Autodesk Fusion 360 part; units mm, degrees
(part 5 of 11)
  line L412 (61.967, 22.9336) -> (61.967, 23.934)
  line L413 (47.167, 19.8345) -> (47.167, 22.9336)
  line L414 (61.967, 19.8345) -> (62.768, 19.8345)
  line L415 (47.967, 23.934) -> (61.967, 23.934)
  line L416 (47.967, 22.9336) -> (47.967, 23.934)
  line L417 (47.967, 22.9336) -> (47.167, 22.9336)
  line L418 (47.167, 19.8345) -> (47.967, 19.8345)
  line L419 (62.768, 22.9336) -> (61.967, 22.9336)
  line L420 (88.162, 4.8841) -> (88.162, 3.8837)
  line L421 (83.685, 14.6338) -> (83.685, 14.0343)
  line L422 (88.961, 3.8837) -> (88.961, 0.7845)
  line L423 (88.162, 3.8837) -> (88.961, 3.8837)
  line L424 (88.162, 0.7845) -> (88.961, 0.7845)
  line L425 (88.162, 3.8837) -> (88.162, 4.8841)
  line L426 (88.961, 0.7845) -> (88.162, 0.7845)
  line L427 (83.685, 14.0343) -> (83.685, 14.6338)
  line L428 (88.961, 3.8837) -> (88.162, 3.8837)
  line L429 (88.961, 0.7845) -> (88.961, 3.8837)
  line L430 (43.205, 95.6582) -> (57.206, 95.6582)
  line L431 (82.162, 10.1634) -> (82.162, 14.6338)
  line L432 (77.137, 9.1836) -> (80.435, 9.1836)
  line L433 (80.435, 10.1634) -> (82.162, 10.1634)
  line L434 (74.161, 3.8837) -> (73.362, 3.8837)
  line L435 (80.435, 9.1836) -> (77.137, 9.1836)
  line L436 (47.681, 62.034) -> (33.68, 62.034)
  line L437 (82.887, 10.9337) -> (82.887, 14.0343)
  line L438 (83.685, 14.6338) -> (82.162, 14.6338)
  line L439 (75.411, 16.4335) -> (75.411, 10.1634)
  line L440 (83.685, 10.9337) -> (83.685, 9.9333)
  line L441 (77.137, 9.1836) -> (77.137, 10.1634)
  line L442 (74.161, 4.8841) -> (74.161, 3.8837)
  line L443 (73.362, 3.8837) -> (74.161, 3.8837)
  line L444 (75.411, 10.1634) -> (75.411, 16.4335)
  line L445 (74.161, 3.8837) -> (74.161, 4.8841)
  line L446 (82.162, 14.6338) -> (82.162, 10.1634)
  line L447 (73.362, 3.8837) -> (73.362, 0.7845)
  line L448 (73.362, 0.7845) -> (74.161, 0.7845)
  line L449 (77.137, 10.1634) -> (77.137, 9.1836)
  line L450 (77.137, 10.1634) -> (75.411, 10.1634)
  line L451 (162.267, 71.1844) -> (162.267, 76.9844)
  line L452 (23.867, 14.0343) -> (24.668, 14.0343)
  line L453 (-118.7201, 61.0336) -> (-118.7201, 62.034)
  line L454 (243.23, 81.084) -> (243.23, 80.0836)
  line L455 (238.979, 80.0836) -> (238.182, 80.0836)
  line L456 (162.267, 99.7592) -> (162.267, 105.5592)
  line L457 (161.467, 96.6592) -> (161.467, 99.7592)
  line L458 (28.117, 10.9337) -> (28.117, 14.0343)
  line L459 (177.068, 68.0838) -> (177.068, 71.1844)
  line L460 (243.23, 76.9844) -> (242.429, 76.9844)
  line L461 (177.068, 71.1844) -> (176.267, 71.1844)
  line L462 (-123.769, 62.034) -> (-123.769, 61.0336)
  line L463 (26.536, 4.8841) -> (26.536, 3.8837)
  line L464 (-123.769, 57.9344) -> (-123.769, 52.1344)
  line L465 (212.856, -9.8664) -> (212.856, -8.8866)
  line L466 (258.029, 76.9844) -> (257.232, 76.9844)
  line L467 (-118.7201, 57.9344) -> (-119.5191, 57.9344)
  line L468 (161.467, 96.6592) -> (162.267, 96.6592)
  line L469 (177.068, 76.9844) -> (177.068, 80.0836)
  line L470 (209.607, -8.1163) -> (209.607, -9.1167)
  line L471 (23.867, 9.9333) -> (23.867, 10.9337)
  line L472 (224.18, 81.084) -> (238.182, 81.084)
  line L473 (-118.7201, 52.1344) -> (-118.7201, 57.9344)
  line L474 (209.607, -4.4162) -> (209.607, -5.0157)
  line L475 (158.018, 99.7592) -> (158.018, 96.6592)
  line L476 (161.467, 108.6602) -> (162.267, 108.6602)
  line L477 (26.536, 3.8837) -> (25.737, 3.8837)
  line L478 (257.232, 81.084) -> (243.23, 81.084)
  line L479 (224.18, 42.984) -> (238.182, 42.984)
  line L480 (210.404, -8.1163) -> (209.607, -8.1163)
  line L481 (-118.7201, 52.1344) -> (-119.5191, 52.1344)
  line L482 (157.217, 105.5592) -> (158.018, 105.5592)
  line L483 (24.668, 14.0343) -> (23.867, 14.0343)
  line L484 (-28.233, 23.934) -> (-14.233, 23.934)
  line L485 (238.979, 80.0836) -> (238.979, 76.9844)
  line L486 (23.867, 10.9337) -> (24.668, 10.9337)
  line L487 (158.018, 105.5592) -> (157.217, 105.5592)
  line L488 (216.154, -9.8664) -> (212.856, -9.8664)
  line L489 (243.23, 80.0836) -> (242.429, 80.0836)
  line L490 (257.232, 71.1844) -> (257.232, 76.9844)
  line L491 (25.737, 0.7845) -> (26.536, 0.7845)
  line L492 (-123.769, 61.0336) -> (-122.97, 61.0336)
  line L493 (-118.7201, 49.0338) -> (-118.7201, 48.0333)
  line L494 (211.131, -4.4162) -> (209.607, -4.4162)
  line L495 (238.182, 76.9844) -> (238.979, 76.9844)
  line L496 (243.23, 76.9844) -> (243.23, 71.1844)
  line L497 (157.217, 96.6592) -> (158.018, 96.6592)
  line L498 (177.068, 80.0836) -> (176.267, 80.0836)
  line L499 (209.607, -8.1163) -> (210.404, -8.1163)
  line L500 (-118.7201, 57.9344) -> (-118.7201, 52.1344)
  line L501 (210.404, -5.0157) -> (209.607, -5.0157)
  line L502 (177.068, 76.9844) -> (176.267, 76.9844)
  line L503 (162.267, 68.0838) -> (162.267, 67.0833)
  line L504 (176.267, 67.0833) -> (176.267, 68.0838)
  line L505 (242.429, 80.0836) -> (242.429, 76.9844)
  line L506 (23.356, 71.1844) -> (23.356, 68.0838)
  line L507 (177.068, 80.0836) -> (177.068, 76.9844)
  line L508 (-122.97, 49.0338) -> (-123.769, 49.0338)
  line L509 (161.467, 105.5592) -> (162.267, 105.5592)
  line L510 (210.404, -8.1163) -> (210.404, -5.0157)
  line L511 (158.018, 105.5592) -> (158.018, 108.6602)
  line L512 (209.607, -9.1167) -> (209.607, -8.1163)
  line L513 (-123.769, 48.0333) -> (-123.769, 49.0338)
  line L514 (258.029, 76.9844) -> (258.029, 80.0836)
  line L515 (158.018, 108.6602) -> (157.217, 108.6602)
  line L516 (238.182, 80.0836) -> (238.979, 80.0836)
  line L517 (24.155, 68.0838) -> (24.155, 67.0833)
  line L518 (-119.5191, 52.1344) -> (-118.7201, 52.1344)
  line L519 (176.267, 76.9844) -> (177.068, 76.9844)
  line L520 (238.979, 76.9844) -> (238.182, 76.9844)
  line L521 (-122.97, 52.1344) -> (-122.97, 49.0338)
  line L522 (176.267, 80.0836) -> (177.068, 80.0836)
  line L523 (210.404, -5.0157) -> (210.404, -8.1163)
  line L524 (24.668, 14.0343) -> (24.668, 10.9337)
  line L525 (177.068, 71.1844) -> (177.068, 68.0838)
  line L526 (242.429, 76.9844) -> (242.429, 80.0836)
  line L527 (162.267, 96.6592) -> (162.267, 95.6582)
  line L528 (211.131, -8.8866) -> (212.856, -8.8866)
  line L529 (24.155, 67.0833) -> (24.155, 68.0838)
  line L530 (212.856, -8.8866) -> (212.856, -9.8664)
  line L531 (-119.5191, 61.0336) -> (-118.7201, 61.0336)
  line L532 (-30.902, 0.1836) -> (8.724, 0.1836)
  line L533 (25.737, 0.7845) -> (25.737, 3.8837)
  line L534 (176.267, 68.0838) -> (176.267, 67.0833)
  line L535 (243.23, 80.0836) -> (243.23, 81.084)
  line L536 (24.155, 71.1844) -> (24.155, 76.9844)
  line L537 (-123.769, 49.0338) -> (-123.769, 48.0333)
  line L538 (23.356, 76.9844) -> (23.356, 80.0836)
  line L539 (258.029, 80.0836) -> (258.029, 76.9844)
  line L540 (-122.97, 52.1344) -> (-123.769, 52.1344)
  line L541 (26.536, 0.7845) -> (25.737, 0.7845)
  line L542 (25.737, 3.8837) -> (26.536, 3.8837)
  line L543 (158.018, 99.7592) -> (157.217, 99.7592)
  line L544 (212.856, -8.8866) -> (211.131, -8.8866)
  line L545 (24.155, 81.084) -> (24.155, 80.0836)
  line L546 (162.267, 108.6602) -> (161.467, 108.6602)
  line L547 (209.607, -4.4162) -> (211.131, -4.4162)
  arc A4 (162.273, 120.9832) -> (160.273, 118.9832) centre (162.273, 118.9832) ccw
  line L548 (-119.5191, 49.0338) -> (-118.7201, 49.0338)
  line L549 (243.23, 71.1844) -> (243.23, 76.9844)
  line L550 (176.267, 68.0838) -> (177.068, 68.0838)
  line L551 (177.068, 68.0838) -> (176.267, 68.0838)
  line L552 (-123.769, 61.0336) -> (-123.769, 62.034)
  line L553 (176.267, 71.1844) -> (177.068, 71.1844)
  line L554 (24.155, 80.0836) -> (24.155, 81.084)
  line L555 (-140.1512, 4.8841) -> (-126.1517, 4.8841)
  line L556 (23.867, 10.9337) -> (23.867, 9.9333)
  line L557 (257.232, 81.084) -> (257.232, 80.0836)
  line L558 (25.737, 3.8837) -> (25.737, 0.7845)
  line L559 (24.155, 68.0838) -> (23.356, 68.0838)
  line L560 (161.467, 108.6602) -> (161.467, 105.5592)
  line L561 (176.267, 80.0836) -> (176.267, 81.084)
  line L562 (209.607, -5.0157) -> (209.607, -4.4162)
  line L563 (24.668, 10.9337) -> (23.867, 10.9337)
  line L564 (157.217, 108.6602) -> (158.018, 108.6602)
  line L565 (176.267, 81.084) -> (176.267, 80.0836)
  line L566 (-118.7201, 61.0336) -> (-119.5191, 61.0336)
  line L567 (28.917, 10.9337) -> (28.117, 10.9337)
  line L568 (176.267, 76.9844) -> (176.267, 71.1844)
  line L569 (162.267, 81.084) -> (176.267, 81.084)
  line L570 (209.607, -5.0157) -> (210.404, -5.0157)
  line L571 (28.117, 14.0343) -> (28.917, 14.0343)
  line L572 (-119.5191, 52.1344) -> (-119.5191, 49.0338)
  line L573 (42.917, 9.9333) -> (28.917, 9.9333)
  line L574 (38.156, 81.084) -> (38.156, 80.0836)
  line L575 (28.917, 10.9337) -> (28.917, 9.9333)
  line L576 (158.018, 96.6592) -> (157.217, 96.6592)
  line L577 (160.273, 118.9832) -> (160.273, 116.1832)
  line L578 (-122.97, 61.0336) -> (-122.97, 57.9344)
  line L579 (157.217, 105.5592) -> (157.217, 99.7592)
  line L580 (-128.5329, 23.934) -> (-142.5325, 23.934)
  line L581 (-118.7201, 49.0338) -> (-119.5191, 49.0338)
  line L582 (38.156, 67.0833) -> (38.156, 68.0838)
  line L583 (176.267, 81.084) -> (162.267, 81.084)
  line L584 (40.537, 4.8841) -> (26.536, 4.8841)
  line L585 (224.18, 9.9333) -> (238.182, 9.9333)
  line L586 (162.267, 108.6602) -> (162.267, 109.6602)
  line L587 (211.131, -8.8866) -> (211.131, -4.4162)
  line L588 (26.536, 4.8841) -> (40.537, 4.8841)
  line L589 (24.155, 71.1844) -> (23.356, 71.1844)
  line L590 (176.267, 71.1844) -> (176.267, 76.9844)
  line L591 (38.156, 67.0833) -> (24.155, 67.0833)
  line L592 (212.856, -9.8664) -> (216.154, -9.8664)
  line L593 (38.156, 68.0838) -> (38.156, 67.0833)
  line L594 (162.267, 96.6592) -> (161.467, 96.6592)
  line L595 (-4.708, 42.984) -> (-18.708, 42.984)
  line L596 (38.156, 76.9844) -> (38.955, 76.9844)
  line L597 (-119.5191, 61.0336) -> (-119.5191, 57.9344)
  line L598 (176.267, 67.0833) -> (162.267, 67.0833)
  line L599 (162.267, 105.5592) -> (161.467, 105.5592)
  line L600 (162.267, 67.0833) -> (176.267, 67.0833)
  line L601 (-122.97, 57.9344) -> (-123.769, 57.9344)
  line L602 (162.267, 99.7592) -> (161.467, 99.7592)
  line L603 (-118.7201, 48.0333) -> (-118.7201, 49.0338)
  line L604 (-118.7201, 62.034) -> (-118.7201, 61.0336)
  line L605 (28.117, 10.9337) -> (28.917, 10.9337)
  line L606 (-123.769, 52.1344) -> (-122.97, 52.1344)
  line L607 (38.156, 80.0836) -> (38.955, 80.0836)
  line L608 (158.018, 96.6592) -> (158.018, 99.7592)
  line L609 (-119.5191, 49.0338) -> (-119.5191, 52.1344)
  line L610 (28.917, 9.9333) -> (28.917, 10.9337)
  line L611 (-123.769, 52.1344) -> (-123.769, 57.9344)
  line L612 (219.132, 48.0333) -> (205.13, 48.0333)
  line L613 (38.955, 80.0836) -> (38.156, 80.0836)
  line L614 (24.155, 81.084) -> (38.156, 81.084)
  line L615 (38.955, 68.0838) -> (38.156, 68.0838)
  line L616 (158.018, 108.6602) -> (158.018, 105.5592)
  line L617 (38.156, 81.084) -> (24.155, 81.084)
  line L618 (28.917, 14.0343) -> (28.117, 14.0343)
  line L619 (-122.97, 49.0338) -> (-122.97, 52.1344)
  line L620 (28.917, 9.9333) -> (42.917, 9.9333)
  line L621 (219.929, 49.0338) -> (219.132, 49.0338)
  line L622 (157.217, 109.6602) -> (157.217, 108.6602)
  line L623 (38.156, 80.0836) -> (38.156, 81.084)
  line L624 (38.156, 71.1844) -> (38.156, 76.9844)
  line L625 (9.867, 23.934) -> (23.867, 23.934)
  line L626 (-109.9941, 80.0836) -> (-109.1951, 80.0836)
  line L627 (200.082, 10.9337) -> (200.879, 10.9337)
  line L628 (219.132, 81.084) -> (205.13, 81.084)
  line L629 (205.13, 14.0343) -> (204.329, 14.0343)
  line L630 (43.205, 71.1844) -> (43.205, 76.9844)
  line L631 (14.342, 42.984) -> (0.342, 42.984)
  line L632 (205.13, 9.9333) -> (205.13, 10.9337)
  line L633 (-109.1951, 80.0836) -> (-109.9941, 80.0836)
  line L634 (223.379, 19.8345) -> (223.379, 22.9336)
  line L635 (200.879, 14.0343) -> (200.879, 10.9337)
  line L636 (43.205, 76.9844) -> (42.406, 76.9844)
  line L637 (223.379, 14.0343) -> (223.379, 10.9337)
  line L638 (205.13, 10.9337) -> (204.329, 10.9337)
  line L639 (-109.9941, 80.0836) -> (-109.9941, 76.9844)
  line L640 (219.929, 14.0343) -> (219.929, 10.9337)
  line L641 (43.205, 80.0836) -> (43.205, 81.084)
  line L642 (42.406, 76.9844) -> (42.406, 80.0836)
  line L643 (205.13, 28.9833) -> (205.13, 29.9838)
  line L644 (219.132, 22.9336) -> (219.929, 22.9336)
  line L645 (-109.1951, 68.0838) -> (-109.9941, 68.0838)
  line L646 (219.929, 80.0836) -> (219.929, 76.9844)
  line L647 (200.879, 38.8844) -> (200.082, 38.8844)
  line L648 (195.605, -5.0157) -> (195.605, -4.4162)
  line L649 (0.342, 42.984) -> (14.342, 42.984)
  line L650 (200.082, 33.0844) -> (200.879, 33.0844)
  line L651 (43.205, 67.0833) -> (43.205, 68.0838)
  line L652 (14.342, 28.9833) -> (0.342, 28.9833)
  line L653 (205.13, 38.8844) -> (204.329, 38.8844)
  line L654 (-109.1951, 76.9844) -> (-109.9941, 76.9844)
  line L655 (200.082, 42.984) -> (186.08, 42.984)
  line L656 (223.379, 10.9337) -> (223.379, 14.0343)
  line L657 (-109.1951, 68.0838) -> (-109.1951, 67.0833)
  line L658 (219.132, 71.1844) -> (219.132, 76.9844)
  line L659 (186.08, 28.9833) -> (200.082, 28.9833)
  line L660 (224.18, 81.084) -> (224.18, 80.0836)
  line L661 (38.955, 80.0836) -> (38.955, 76.9844)
  line L662 (42.406, 80.0836) -> (43.205, 80.0836)
  line L663 (219.132, 76.9844) -> (219.132, 71.1844)
  line L664 (219.132, 80.0836) -> (219.929, 80.0836)
  line L665 (157.217, 68.0838) -> (158.018, 68.0838)
  line L666 (204.329, 14.0343) -> (204.329, 10.9337)
  line L667 (-109.1951, 71.1844) -> (-109.1951, 76.9844)
  line L668 (200.082, 14.0343) -> (200.879, 14.0343)
  line L669 (200.879, 10.9337) -> (200.879, 14.0343)
  line L670 (205.13, 23.934) -> (219.132, 23.934)
  line L671 (205.13, 9.9333) -> (219.132, 9.9333)
  line L672 (219.132, 23.934) -> (205.13, 23.934)
  line L673 (195.605, 4.8841) -> (195.605, 3.8837)
  line L674 (-109.9941, 68.0838) -> (-109.1951, 68.0838)
  line L675 (219.132, 9.9333) -> (205.13, 9.9333)
  line L676 (200.082, 28.9833) -> (186.08, 28.9833)
  line L677 (-109.9941, 76.9844) -> (-109.9941, 80.0836)
  line L678 (204.329, 10.9337) -> (204.329, 14.0343)
  line L679 (158.018, 68.0838) -> (158.018, 71.1844)
  line L680 (-109.1951, 67.0833) -> (-109.1951, 68.0838)
  line L681 (-114.244, 109.6602) -> (-128.2451, 109.6602)
  line L682 (-142.5325, 9.9333) -> (-128.5329, 9.9333)
  line L683 (219.132, 76.9844) -> (219.929, 76.9844)
  line L684 (186.08, 42.984) -> (200.082, 42.984)
  line L685 (219.929, 76.9844) -> (219.929, 80.0836)
  line L686 (224.18, 80.0836) -> (224.18, 81.084)
  line L687 (195.605, 4.8841) -> (209.607, 4.8841)
  line L688 (195.605, -9.1167) -> (195.605, -8.1163)
  line L689 (158.018, 76.9844) -> (158.018, 80.0836)
  line L690 (238.182, 81.084) -> (238.182, 80.0836)
  line L691 (157.217, 67.0833) -> (157.217, 68.0838)
  line L692 (-95.194, 76.9844) -> (-94.395, 76.9844)
  line L693 (-94.395, 80.0836) -> (-95.194, 80.0836)
  line L694 (205.13, 10.9337) -> (205.13, 9.9333)
  line L695 (161.467, 71.1844) -> (161.467, 68.0838)
  line L696 (200.879, 14.0343) -> (200.082, 14.0343)
  line L697 (224.18, -9.1167) -> (238.182, -9.1167)
  line L698 (-109.9941, 71.1844) -> (-109.1951, 71.1844)
  line L699 (158.018, 71.1844) -> (157.217, 71.1844)
  line L700 (157.217, 81.084) -> (157.217, 80.0836)
  line L701 (-94.395, 71.1844) -> (-95.194, 71.1844)
  line L702 (224.18, 80.0836) -> (223.379, 80.0836)
  line L703 (219.132, 80.0836) -> (219.132, 81.084)
  line L704 (186.08, 9.9333) -> (200.082, 9.9333)
  line L705 (224.18, 76.9844) -> (223.379, 76.9844)
  line L706 (157.217, 68.0838) -> (157.217, 67.0833)
  line L707 (162.267, 81.084) -> (162.267, 80.0836)
  line L708 (-95.194, 67.0833) -> (-109.1951, 67.0833)
  line L709 (204.329, 10.9337) -> (205.13, 10.9337)
  line L710 (200.082, 9.9333) -> (186.08, 9.9333)
  line L711 (158.018, 76.9844) -> (157.217, 76.9844)
  line L712 (-95.194, 81.084) -> (-95.194, 80.0836)
  line L713 (161.467, 80.0836) -> (161.467, 76.9844)
  line L714 (-109.1951, 67.0833) -> (-95.194, 67.0833)
  line L715 (223.379, 76.9844) -> (224.18, 76.9844)
  line L716 (223.379, 80.0836) -> (224.18, 80.0836)
  line L717 (162.267, 80.0836) -> (161.467, 80.0836)
  line L718 (238.182, 76.9844) -> (238.182, 71.1844)
  line L719 (-95.194, 71.1844) -> (-94.395, 71.1844)
  line L720 (219.929, 80.0836) -> (219.132, 80.0836)
  line L721 (-95.194, 71.1844) -> (-95.194, 76.9844)
  line L722 (42.917, 10.9337) -> (43.718, 10.9337)
  line L723 (161.467, 76.9844) -> (162.267, 76.9844)
  line L724 (219.929, 76.9844) -> (219.132, 76.9844)
  line L725 (210.404, 0.7845) -> (209.607, 0.7845)
  line L726 (205.13, 81.084) -> (219.132, 81.084)
  line L727 (-95.194, 68.0838) -> (-94.395, 68.0838)
  line L728 (-94.395, 68.0838) -> (-95.194, 68.0838)
  line L729 (224.567, 118.9832) -> (224.567, 116.1832)
  line L730 (-95.194, 81.084) -> (-109.1951, 81.084)
  line L731 (209.607, 3.8837) -> (209.607, 4.8841)
  line L732 (162.267, 76.9844) -> (161.467, 76.9844)
  line L733 (224.18, 71.1844) -> (224.18, 76.9844)
  line L734 (162.267, 76.9844) -> (162.267, 71.1844)
  line L735 (41.336, 3.8837) -> (40.537, 3.8837)
  circle A5 centre (236.267, 117.5832) radius 1.7
  line L736 (210.404, 0.7845) -> (210.404, 3.8837)
  line L737 (41.336, 0.7845) -> (40.537, 0.7845)
  line L738 (23.356, 80.0836) -> (24.155, 80.0836)
  line L739 (249.967, 114.1832) -> (261.656, 114.1832)
  line L740 (212.856, 3.4138) -> (211.131, 3.4138)
  line L741 (157.217, 71.1844) -> (157.217, 76.9844)
  line L742 (40.537, 3.8837) -> (41.336, 3.8837)
  line L743 (-95.194, 80.0836) -> (-94.395, 80.0836)
  line L744 (-95.194, 67.0833) -> (-95.194, 68.0838)
  line L745 (238.182, 71.1844) -> (238.182, 76.9844)
  arc A6 (222.567, 114.1832) -> (224.567, 116.1832) centre (222.567, 116.1832) ccw
  line L746 (157.217, 80.0836) -> (157.217, 81.084)
  line L747 (43.718, 14.0343) -> (43.718, 10.9337)
  line L748 (224.18, 76.9844) -> (224.18, 71.1844)
  line L749 (211.131, 3.4138) -> (211.131, 0.1836)
  line L750 (-95.194, 68.0838) -> (-95.194, 67.0833)
  line L751 (41.336, 0.7845) -> (41.336, 3.8837)
  line L752 (-109.1951, 81.084) -> (-95.194, 81.084)
  line L753 (23.356, 76.9844) -> (24.155, 76.9844)
  line L754 (40.537, 4.8841) -> (40.537, 3.8837)
  line L755 (-95.194, 76.9844) -> (-95.194, 71.1844)
  line L756 (210.404, 3.8837) -> (209.607, 3.8837)
  line L757 (161.467, 71.1844) -> (162.267, 71.1844)
  line L758 (42.917, 9.9333) -> (42.917, 10.9337)
  line L759 (-95.194, 80.0836) -> (-95.194, 81.084)
  line L760 (236.667, 120.9832) -> (235.867, 120.9832)
  line L761 (247.967, 118.9832) -> (247.967, 116.1832)
  line L762 (219.132, 81.084) -> (219.132, 80.0836)
  line L763 (209.607, 0.1836) -> (211.131, 0.1836)
  line L764 (223.379, 76.9844) -> (223.379, 80.0836)
  arc A7 (226.567, 120.9832) -> (224.567, 118.9832) centre (226.567, 118.9832) ccw
  line L765 (43.718, 14.0343) -> (42.917, 14.0343)
  line L766 (223.379, 80.0836) -> (223.379, 76.9844)
  line L767 (161.467, 68.0838) -> (161.467, 71.1844)
  line L768 (161.467, 76.9844) -> (161.467, 80.0836)
  line L769 (212.856, 4.3343) -> (212.856, 3.4138)
  line L770 (158.018, 68.0838) -> (157.217, 68.0838)
  line L771 (212.856, 3.4138) -> (212.856, 4.3343)
  line L772 (-94.395, 76.9844) -> (-95.194, 76.9844)
  arc A8 (247.967, 118.9832) -> (245.967, 120.9832) centre (245.967, 118.9832) ccw
  line L773 (209.607, 4.8841) -> (209.607, 3.8837)
  line L774 (161.467, 68.0838) -> (162.267, 68.0838)
  line L775 (43.718, 10.9337) -> (43.718, 14.0343)
  line L776 (209.607, 0.1836) -> (209.607, 0.7845)
  line L777 (23.356, 80.0836) -> (23.356, 76.9844)
  line L778 (41.336, 3.8837) -> (41.336, 0.7845)
  line L779 (176.267, 109.6602) -> (162.267, 109.6602)
  line L780 (157.217, 76.9844) -> (158.018, 76.9844)
  line L781 (210.404, 3.8837) -> (210.404, 0.7845)
  line L782 (162.267, 67.0833) -> (162.267, 68.0838)
  line L783 (209.607, 0.7845) -> (209.607, 0.1836)
  line L784 (40.537, 0.7845) -> (41.336, 0.7845)
  line L785 (209.607, 0.7845) -> (210.404, 0.7845)
  circle A9 centre (236.267, 117.5832) radius 1.7
  line L786 (162.267, 68.0838) -> (161.467, 68.0838)
  line L787 (211.131, 3.4138) -> (212.856, 3.4138)
  line L788 (158.018, 80.0836) -> (158.018, 76.9844)
  arc A10 (247.967, 116.1832) -> (249.967, 114.1832) centre (249.967, 116.1832) ccw
  line L789 (162.267, 80.0836) -> (162.267, 81.084)
  line L790 (212.856, 4.3343) -> (216.154, 4.3343)
  line L791 (23.356, 68.0838) -> (24.155, 68.0838)
  line L792 (157.217, 80.0836) -> (158.018, 80.0836)
  line L793 (40.537, 3.8837) -> (40.537, 4.8841)
  line L794 (245.967, 120.9832) -> (226.567, 120.9832)
  line L795 (-23.47, 48.0333) -> (-9.469, 48.0333)
  line L796 (-81.201, 114.1832) -> (5.398, 114.1832)
  line L797 (176.267, 95.6582) -> (162.267, 95.6582)
  line L798 (23.356, 68.0838) -> (23.356, 71.1844)
  line L799 (157.217, 76.9844) -> (157.217, 71.1844)
  line L800 (42.917, 14.0343) -> (43.718, 14.0343)
  line L801 (162.267, 109.6602) -> (162.267, 108.6602)
  line L802 (24.155, 80.0836) -> (23.356, 80.0836)
  line L803 (209.607, 3.8837) -> (210.404, 3.8837)
  line L804 (158.018, 71.1844) -> (158.018, 68.0838)
  line L805 (158.018, 80.0836) -> (157.217, 80.0836)
  line L806 (211.131, 0.1836) -> (211.131, 3.4138)
  line L807 (211.131, 0.1836) -> (209.607, 0.1836)
  line L808 (24.155, 76.9844) -> (23.356, 76.9844)
  line L809 (161.467, 80.0836) -> (162.267, 80.0836)
  line L810 (157.217, 71.1844) -> (158.018, 71.1844)
  line L811 (42.917, 10.9337) -> (42.917, 9.9333)
  line L812 (43.718, 10.9337) -> (42.917, 10.9337)
  line L813 (216.154, 4.3343) -> (212.856, 4.3343)
  line L814 (161.467, 99.7592) -> (161.467, 96.6592)
  line L815 (23.356, 71.1844) -> (24.155, 71.1844)
  line L816 (224.18, 28.9833) -> (238.182, 28.9833)
  line L817 (157.217, 108.6602) -> (157.217, 109.6602)
  line L818 (242.429, 80.0836) -> (243.23, 80.0836)
  line L819 (24.155, 76.9844) -> (24.155, 71.1844)
  line L820 (162.267, 71.1844) -> (161.467, 71.1844)
  line L821 (243.23, 81.084) -> (257.232, 81.084)
  line L822 (157.217, 99.7592) -> (158.018, 99.7592)
  line L823 (242.429, 76.9844) -> (243.23, 76.9844)
  line L824 (157.217, 99.7592) -> (157.217, 105.5592)
  line L825 (162.267, 105.5592) -> (162.267, 99.7592)
  line L826 (-119.5191, 57.9344) -> (-118.7201, 57.9344)
  line L827 (28.117, 14.0343) -> (28.117, 10.9337)
  line L828 (161.467, 99.7592) -> (162.267, 99.7592)
  line L829 (257.232, 76.9844) -> (258.029, 76.9844)
  line L830 (-128.2451, 95.6582) -> (-114.244, 95.6582)
  line L831 (257.232, 80.0836) -> (257.232, 81.084)
  line L832 (157.217, 95.6582) -> (157.217, 96.6592)
  line L833 (257.232, 80.0836) -> (258.029, 80.0836)
  line L834 (238.182, 81.084) -> (224.18, 81.084)
  line L835 (238.182, 28.9833) -> (224.18, 28.9833)
  line L836 (257.232, 76.9844) -> (257.232, 71.1844)
  arc A11 (158.273, 114.1832) -> (160.273, 116.1832) centre (158.273, 116.1832) ccw
  line L837 (161.467, 105.5592) -> (161.467, 108.6602)
  line L838 (24.668, 10.9337) -> (24.668, 14.0343)
  line L839 (157.217, 96.6592) -> (157.217, 95.6582)
  line L840 (162.267, 95.6582) -> (162.267, 96.6592)
  line L841 (-122.97, 57.9344) -> (-122.97, 61.0336)
  line L842 (-123.769, 57.9344) -> (-122.97, 57.9344)
  line L843 (238.979, 76.9844) -> (238.979, 80.0836)
  line L844 (238.182, 80.0836) -> (238.182, 81.084)
  line L845 (26.536, 3.8837) -> (26.536, 4.8841)
  line L846 (-119.5191, 57.9344) -> (-119.5191, 61.0336)
  line L847 (258.029, 80.0836) -> (257.232, 80.0836)
  line L848 (211.131, -4.4162) -> (211.131, -8.8866)
  line L849 (88.162, -8.1163) -> (88.961, -8.1163)
  arc A12 (88.274, -18.7426) -> (90.274, -20.7426) centre (90.274, -18.7426) ccw
  line L850 (88.162, 0.7845) -> (88.162, -5.0157)
  line L851 (74.161, -9.1167) -> (74.161, -8.1163)
  line L852 (88.961, -5.0157) -> (88.961, -8.1163)
  line L853 (74.161, -8.1163) -> (73.362, -8.1163)
  line L854 (73.362, -5.0157) -> (74.161, -5.0157)
  line L855 (74.161, -8.1163) -> (74.161, -9.1167)
  line L856 (74.161, -9.1167) -> (88.162, -9.1167)
  line L857 (73.362, -8.1163) -> (73.362, -5.0157)
  line L858 (88.961, -5.0157) -> (88.162, -5.0157)
  line L859 (88.162, -8.1163) -> (88.162, -9.1167)
  line L860 (73.362, -8.1163) -> (74.161, -8.1163)
  arc A13 (88.274, -15.9426) -> (86.274, -13.9426) centre (86.274, -15.9426) ccw
  line L861 (88.162, -9.1167) -> (74.161, -9.1167)
  line L862 (73.362, -5.0157) -> (73.362, -8.1163)
  line L863 (88.961, -8.1163) -> (88.961, -5.0157)
  line L864 (88.961, -8.1163) -> (88.162, -8.1163)
  line L865 (88.162, -5.0157) -> (88.961, -5.0157)
  line L866 (88.162, -5.0157) -> (88.162, 0.7845)
  line L867 (88.162, -9.1167) -> (88.162, -8.1163)
  line L868 (74.161, -5.0157) -> (73.362, -5.0157)
  line L869 (74.161, -5.0157) -> (74.161, 0.7845)
  line L870 (74.161, 0.7845) -> (74.161, -5.0157)
  line L871 (88.274, -18.7426) -> (88.274, -15.9426)
  line L872 (47.967, 10.9337) -> (47.967, 9.9333)
  line L873 (50.349, 3.8837) -> (50.349, 4.8841)
  line L874 (64.348, 4.8841) -> (64.348, 3.8837)
  line L875 (61.967, 14.0343) -> (62.768, 14.0343)
  line L876 (47.167, 14.0343) -> (47.167, 10.9337)
  line L877 (49.548, 3.8837) -> (50.349, 3.8837)
  line L878 (65.149, 3.8837) -> (64.348, 3.8837)
  line L879 (64.348, 3.8837) -> (64.348, 4.8841)
  line L880 (62.768, 14.0343) -> (62.768, 10.9337)
  line L881 (47.967, 14.0343) -> (47.167, 14.0343)
  line L882 (47.167, 10.9337) -> (47.967, 10.9337)
  line L883 (47.167, 10.9337) -> (47.167, 14.0343)
  line L884 (64.348, 3.8837) -> (65.149, 3.8837)
  line L885 (50.349, 4.8841) -> (50.349, 3.8837)
  line L886 (47.967, 9.9333) -> (47.967, 10.9337)
  line L887 (61.967, 10.9337) -> (61.967, 9.9333)
  line L888 (47.967, 10.9337) -> (47.167, 10.9337)
  line L889 (61.967, 9.9333) -> (47.967, 9.9333)
  line L890 (61.967, 9.9333) -> (61.967, 10.9337)
  line L891 (62.768, 10.9337) -> (62.768, 14.0343)
  line L892 (64.348, 4.8841) -> (50.349, 4.8841)
  line L893 (50.349, 4.8841) -> (64.348, 4.8841)
  line L894 (47.167, 14.0343) -> (47.967, 14.0343)
  line L895 (61.967, 10.9337) -> (62.768, 10.9337)
  line L896 (62.768, 14.0343) -> (61.967, 14.0343)
  line L897 (62.768, 10.9337) -> (61.967, 10.9337)
  line L898 (50.349, 3.8837) -> (49.548, 3.8837)
  line L899 (47.967, 9.9333) -> (61.967, 9.9333)
  line L900 (-94.9076, 28.9833) -> (-80.9079, 28.9833)
  line L901 (123.367, 61.0336) -> (123.367, 57.9344)
  line L902 (-85.6704, 62.034) -> (-99.6701, 62.034)
  line L903 (157.217, 23.934) -> (143.217, 23.934)
  line L904 (158.273, -13.9426) -> (113.674, -13.9426)
  line L905 (157.217, 4.8841) -> (143.217, 4.8841)
  line L906 (-76.144, 81.084) -> (-90.1451, 81.084)
  line L907 (-80.9079, 28.9833) -> (-94.9076, 28.9833)
  line L908 (157.217, 81.084) -> (143.217, 81.084)
  line L909 (157.217, 48.0333) -> (143.217, 48.0333)
  line L910 (157.217, 62.034) -> (143.217, 62.034)
  line L911 (124.167, 61.0336) -> (123.367, 61.0336)
  line L912 (123.367, 52.1344) -> (124.167, 52.1344)
  line L913 (-80.9079, 42.984) -> (-94.9076, 42.984)
  line L914 (143.217, 48.0333) -> (157.217, 48.0333)
  line L915 (123.367, 49.0338) -> (123.367, 52.1344)
  line L916 (124.167, 57.9344) -> (124.167, 52.1344)
  line L917 (-99.6701, 48.0333) -> (-85.6704, 48.0333)
  line L918 (157.217, 95.6582) -> (143.217, 95.6582)
  line L919 (143.217, 67.0833) -> (157.217, 67.0833)
  line L920 (123.367, 49.0338) -> (124.167, 49.0338)
  line L921 (143.217, 23.934) -> (157.217, 23.934)
  line L922 (143.217, 109.6602) -> (157.217, 109.6602)
  line L923 (-76.144, 67.0833) -> (-90.1451, 67.0833)
  line L924 (143.217, 95.6582) -> (157.217, 95.6582)
  line L925 (143.217, 81.084) -> (157.217, 81.084)
  line L926 (113.674, 114.1832) -> (158.273, 114.1832)
  line L927 (157.217, 9.9333) -> (143.217, 9.9333)
  line L928 (143.217, 62.034) -> (157.217, 62.034)
  line L929 (143.217, 9.9333) -> (157.217, 9.9333)
  line L930 (-86.2521, -9.8664) -> (-89.551, -9.8664)
  line L931 (123.367, 57.9344) -> (124.167, 57.9344)
  line L932 (157.217, 67.0833) -> (143.217, 67.0833)
  line L933 (123.367, 57.9344) -> (123.367, 61.0336)
  line L934 (124.167, 49.0338) -> (123.367, 49.0338)
  line L935 (-89.551, 4.3343) -> (-86.2521, 4.3343)
  line L936 (124.167, 49.0338) -> (124.167, 48.0333)
  line L937 (123.367, 52.1344) -> (123.367, 49.0338)
  line L938 (107.274, 52.509) -> (107.274, 54.0334)
  line L939 (143.217, 62.034) -> (143.217, 61.0336)
  line L940 (124.167, 99.7592) -> (124.167, 105.5592)
  line L941 (110.974, 52.509) -> (111.973, 52.509)
  line L942 (124.167, 105.5592) -> (123.367, 105.5592)
  line L943 (123.367, 96.6592) -> (124.167, 96.6592)
  line L944 (71.78, 48.0333) -> (71.78, 49.0338)
  line L945 (123.367, 105.5592) -> (123.367, 108.6602)
  line L946 (95.306, 99.7592) -> (95.306, 105.5592)
  line L947 (85.781, 49.0338) -> (86.58, 49.0338)
  line L948 (124.167, 99.7592) -> (123.367, 99.7592)
  line L949 (86.58, 49.0338) -> (85.781, 49.0338)
  line L950 (124.167, 76.9844) -> (124.167, 71.1844)
  line L951 (138.167, 109.6602) -> (138.167, 108.6602)
  line L952 (111.423, 59.0591) -> (111.423, 55.7585)
  line L953 (138.167, 48.0333) -> (138.167, 49.0338)
  line L954 (107.874, 52.509) -> (107.274, 52.509)
  line L955 (86.58, 49.0338) -> (86.58, 52.1344)
  line L956 (100.355, 95.6582) -> (100.355, 96.6592)
  line L957 (85.781, 49.0338) -> (85.781, 48.0333)
  line L958 (114.356, 105.5592) -> (114.356, 99.7592)
  line L959 (138.968, 49.0338) -> (138.968, 52.1344)
  line L960 (123.367, 108.6602) -> (124.167, 108.6602)
  line L961 (123.367, 108.6602) -> (123.367, 105.5592)
  line L962 (96.105, 96.6592) -> (95.306, 96.6592)
  line L963 (138.968, 61.0336) -> (138.167, 61.0336)
  line L964 (99.556, 96.6592) -> (100.355, 96.6592)
  line L965 (71.78, 57.9344) -> (71.78, 52.1344)
  line L966 (123.367, 96.6592) -> (123.367, 99.7592)
  line L967 (138.968, 49.0338) -> (138.167, 49.0338)
  line L968 (142.417, 57.9344) -> (142.417, 61.0336)
  line L969 (124.167, 80.0836) -> (124.167, 81.084)
  line L970 (114.356, 96.6592) -> (114.356, 95.6582)
  line L971 (110.974, 53.3084) -> (107.874, 53.3084)
  line L972 (124.167, 108.6602) -> (123.367, 108.6602)
  line L973 (142.417, 52.1344) -> (143.217, 52.1344)
  line L974 (38.442, 38.8844) -> (38.442, 33.0844)
  line L975 (138.167, 71.1844) -> (138.167, 76.9844)
  line L976 (138.167, 57.9344) -> (138.968, 57.9344)
  line L977 (100.355, 99.7592) -> (100.355, 105.5592)
  line L978 (86.58, 57.9344) -> (85.781, 57.9344)
  line L979 (86.58, 61.0336) -> (86.58, 57.9344)
  line L980 (124.167, 95.6582) -> (124.167, 96.6592)
  line L981 (95.306, 96.6592) -> (96.105, 96.6592)
  line L982 (124.167, 108.6602) -> (124.167, 109.6602)
  line L983 (99.556, 99.7592) -> (99.556, 96.6592)
  line L984 (123.367, 80.0836) -> (124.167, 80.0836)
  line L985 (85.781, 52.1344) -> (86.58, 52.1344)
  line L986 (86.58, 52.1344) -> (85.781, 52.1344)
  line L987 (86.58, 61.0336) -> (85.781, 61.0336)
  line L988 (124.167, 109.6602) -> (124.167, 108.6602)
  line L989 (142.417, 61.0336) -> (142.417, 57.9344)
  line L990 (64.348, -5.0157) -> (64.348, 0.7845)
  line L991 (65.149, -5.0157) -> (65.149, -8.1163)
  line L992 (50.349, -5.0157) -> (49.548, -5.0157)
  line L993 (50.349, -9.1167) -> (64.348, -9.1167)
  line L994 (65.149, 0.7845) -> (65.149, 3.8837)
  line L995 (64.348, 0.7845) -> (64.348, -5.0157)
  line L996 (65.149, 0.7845) -> (64.348, 0.7845)
  line L997 (49.548, -8.1163) -> (50.349, -8.1163)
  line L998 (50.349, -5.0157) -> (50.349, 0.7845)
  line L999 (65.149, -8.1163) -> (65.149, -5.0157)
  line L1000 (50.349, 0.7845) -> (50.349, -5.0157)
  line L1001 (50.349, -9.1167) -> (50.349, -8.1163)
  line L1002 (49.548, -8.1163) -> (49.548, -5.0157)
  line L1003 (65.149, -8.1163) -> (64.348, -8.1163)
  line L1004 (49.548, 0.7845) -> (50.349, 0.7845)
  line L1005 (49.548, 3.8837) -> (49.548, 0.7845)
  line L1006 (64.348, -9.1167) -> (50.349, -9.1167)
  line L1007 (50.349, -8.1163) -> (49.548, -8.1163)
  line L1008 (64.348, -8.1163) -> (64.348, -9.1167)
  line L1009 (49.548, 0.7845) -> (49.548, 3.8837)
  line L1010 (50.349, 0.7845) -> (49.548, 0.7845)
  line L1011 (64.348, 0.7845) -> (65.149, 0.7845)
  line L1012 (65.149, -5.0157) -> (64.348, -5.0157)
  line L1013 (49.548, -5.0157) -> (50.349, -5.0157)
  line L1014 (64.348, -9.1167) -> (64.348, -8.1163)
  line L1015 (50.349, -8.1163) -> (50.349, -9.1167)
  line L1016 (64.348, -5.0157) -> (65.149, -5.0157)
  line L1017 (43.205, 109.6602) -> (57.206, 109.6602)
  line L1018 (49.548, -5.0157) -> (49.548, -8.1163)
  line L1019 (64.348, -8.1163) -> (65.149, -8.1163)
  line L1020 (33.68, 48.0333) -> (47.681, 48.0333)
  line L1021 (65.149, 3.8837) -> (65.149, 0.7845)
  line L1022 (38.442, 28.9833) -> (52.442, 28.9833)
  line L1023 (57.206, 95.6582) -> (43.205, 95.6582)
  line L1024 (57.206, 67.0833) -> (43.205, 67.0833)
  line L1025 (43.205, 67.0833) -> (57.206, 67.0833)
  line L1026 (124.167, 61.0336) -> (124.167, 62.034)
  line L1027 (-94.9076, 42.984) -> (-80.9079, 42.984)
  line L1028 (143.217, -9.1167) -> (157.217, -9.1167)
  line L1029 (138.167, 49.0338) -> (138.167, 48.0333)
  line L1030 (124.167, 48.0333) -> (124.167, 49.0338)
  line L1031 (-90.1451, 81.084) -> (-76.144, 81.084)
  line L1032 (157.217, -9.1167) -> (143.217, -9.1167)
  line L1033 (138.167, 52.1344) -> (138.167, 57.9344)
  line L1034 (123.367, 61.0336) -> (124.167, 61.0336)
  line L1035 (-89.551, -9.8664) -> (-86.2521, -9.8664)
  line L1036 (124.167, 52.1344) -> (123.367, 52.1344)
  line L1037 (-90.1451, 67.0833) -> (-76.144, 67.0833)
  line L1038 (124.167, 57.9344) -> (123.367, 57.9344)
  line L1039 (143.217, 4.8841) -> (157.217, 4.8841)
  line L1040 (124.167, 52.1344) -> (124.167, 57.9344)
  line L1041 (-85.6704, 48.0333) -> (-99.6701, 48.0333)
  line L1042 (124.167, 62.034) -> (124.167, 61.0336)
  line L1043 (157.217, 109.6602) -> (143.217, 109.6602)
  line L1044 (-76.144, 95.6582) -> (-90.1451, 95.6582)
  arc A14 (111.674, 116.1832) -> (113.674, 114.1832) centre (113.674, 116.1832) ccw
  circle A15 centre (99.974, 117.5832) radius 1.7
  line L1045 (143.217, 80.0836) -> (142.417, 80.0836)
  line L1046 (90.83, 71.7838) -> (90.83, 71.1844)
  line L1047 (28.917, 19.8345) -> (28.117, 19.8345)
  line L1048 (162.273, -20.7426) -> (181.673, -20.7426)
  line L1049 (99.556, 105.5592) -> (100.355, 105.5592)
  line L1050 (143.217, 80.0836) -> (143.217, 81.084)
  line L1051 (80.506, 105.5592) -> (80.506, 108.6602)
  line L1052 (28.117, 19.8345) -> (28.917, 19.8345)
  line L1053 (102.073, 53.3084) -> (98.973, 53.3084)
  line L1054 (28.117, 22.9336) -> (28.117, 19.8345)
  line L1055 (89.306, 71.7838) -> (90.83, 71.7838)
  line L1056 (98.204, 60.7841) -> (98.204, 59.0591)
  arc A16 (160.273, -18.7426) -> (162.273, -20.7426) centre (162.273, -18.7426) ccw
  line L1057 (42.917, 23.934) -> (28.917, 23.934)
  line L1058 (143.217, 71.1844) -> (143.217, 76.9844)
  line L1059 (90.83, 71.1844) -> (90.031, 71.1844)
  line L1060 (142.417, 76.9844) -> (142.417, 80.0836)
  line L1061 (138.167, 105.5592) -> (138.167, 99.7592)
  line L1062 (102.673, 54.0334) -> (102.673, 52.509)
  line L1063 (80.506, 96.6592) -> (80.506, 99.7592)
  line L1064 (142.417, 96.6592) -> (142.417, 99.7592)
  line L1065 (81.305, 105.5592) -> (80.506, 105.5592)
  line L1066 (102.073, 52.509) -> (102.673, 52.509)
  line L1067 (115.155, 105.5592) -> (114.356, 105.5592)
  line L1068 (138.968, 105.5592) -> (138.167, 105.5592)
  line L1069 (138.968, 99.7592) -> (138.968, 96.6592)
  circle A17 centre (236.267, -17.3426) radius 1.7
  line L1070 (247.967, -18.7426) -> (247.967, -15.9426)
  line L1071 (90.83, 68.0838) -> (90.031, 68.0838)
  line L1072 (95.306, 109.6602) -> (81.305, 109.6602)
  line L1073 (97.224, 55.7585) -> (98.204, 55.7585)
  line L1074 (76.256, 99.7592) -> (77.055, 99.7592)
  line L1075 (138.968, 105.5592) -> (138.968, 108.6602)
  line L1076 (138.968, 68.0838) -> (138.167, 68.0838)
  line L1077 (143.217, 96.6592) -> (142.417, 96.6592)
  line L1078 (114.356, 109.6602) -> (114.356, 108.6602)
  line L1079 (224.567, -18.7426) -> (224.567, -15.9426)
  line L1080 (143.217, 76.9844) -> (143.217, 71.1844)
  line L1081 (143.217, 105.5592) -> (143.217, 99.7592)
  line L1082 (87.581, 67.3134) -> (89.306, 67.3134)
  line L1083 (143.217, 67.0833) -> (143.217, 68.0838)
  line L1084 (76.256, 67.0833) -> (62.255, 67.0833)
  line L1085 (28.117, 19.8345) -> (28.117, 22.9336)
  line L1086 (142.417, 105.5592) -> (142.417, 108.6602)
  line L1087 (115.155, 105.5592) -> (115.155, 108.6602)
  line L1088 (43.718, 19.8345) -> (43.718, 22.9336)
  line L1089 (99.556, 108.6602) -> (99.556, 105.5592)
  circle A18 centre (236.267, -17.3426) radius 1.7
  line L1090 (42.917, 22.9336) -> (43.718, 22.9336)
  line L1091 (76.256, 105.5592) -> (77.055, 105.5592)
  line L1092 (102.073, 53.3084) -> (102.073, 52.509)
  arc A19 (249.967, -13.9426) -> (247.967, -15.9426) centre (249.967, -15.9426) ccw
  line L1093 (98.204, 54.0334) -> (98.204, 55.7585)
  line L1094 (81.305, 109.6602) -> (95.306, 109.6602)
  line L1095 (28.917, 23.934) -> (42.917, 23.934)
  line L1096 (98.204, 60.7841) -> (104.474, 60.7841)
  line L1097 (138.167, 80.0836) -> (138.167, 81.084)
  line L1098 (76.256, 109.6602) -> (76.256, 108.6602)
  line L1099 (-104.601, -20.7426) -> (-85.201, -20.7426)
  arc A20 (111.674, 118.9832) -> (109.674, 120.9832) centre (109.674, 118.9832) ccw
  circle A21 centre (171.973, -17.3426) radius 1.7
  line L1100 (98.204, 54.0334) -> (102.673, 54.0334)
  line L1101 (98.204, 55.7585) -> (98.204, 54.0334)
  line L1102 (226.567, -20.7426) -> (245.967, -20.7426)
  line L1103 (76.256, 108.6602) -> (77.055, 108.6602)
  line L1104 (142.417, 108.6602) -> (142.417, 105.5592)
  line L1105 (160.273, -18.7426) -> (160.273, -15.9426)
  line L1106 (261.656, -13.9426) -> (249.967, -13.9426)
  line L1107 (28.917, 22.9336) -> (28.917, 23.934)
  line L1108 (142.417, 76.9844) -> (143.217, 76.9844)
  line L1109 (143.217, 105.5592) -> (142.417, 105.5592)
  line L1110 (102.673, 54.0334) -> (98.204, 54.0334)
  line L1111 (138.968, 76.9844) -> (138.167, 76.9844)
  line L1112 (76.256, 96.6592) -> (76.256, 95.6582)
  line L1113 (103.374, 117.1832) -> (103.374, 117.9832)
  line L1114 (138.167, 108.6602) -> (138.167, 109.6602)
  line L1115 (102.073, 52.509) -> (102.073, 53.3084)
  line L1116 (138.167, 99.7592) -> (138.968, 99.7592)
  arc A22 (185.673, -13.9426) -> (183.673, -15.9426) centre (185.673, -15.9426) ccw
  line L1117 (235.867, -20.7426) -> (236.667, -20.7426)
  line L1118 (62.255, 109.6602) -> (76.256, 109.6602)
  line L1119 (143.217, 99.7592) -> (142.417, 99.7592)
  line L1120 (62.255, 108.6602) -> (62.255, 109.6602)
  line L1121 (77.055, 96.6592) -> (77.055, 99.7592)
  line L1122 (97.224, 59.0591) -> (98.204, 59.0591)
  line L1123 (138.167, 108.6602) -> (138.968, 108.6602)
  arc A23 (224.567, -15.9426) -> (222.567, -13.9426) centre (222.567, -15.9426) ccw
  line L1124 (-99.6701, 62.034) -> (-85.6704, 62.034)
  line L1125 (142.417, 108.6602) -> (143.217, 108.6602)
  line L1126 (62.255, 99.7592) -> (62.255, 105.5592)
  line L1127 (62.255, 81.084) -> (76.256, 81.084)
  line L1128 (97.224, 55.7585) -> (97.224, 59.0591)
  line L1129 (142.417, 99.7592) -> (143.217, 99.7592)
  line L1130 (62.255, 96.6592) -> (62.255, 95.6582)
  line L1131 (-90.1451, 109.6602) -> (-76.144, 109.6602)
  line L1132 (87.581, 79.6137) -> (89.306, 79.6137)
  line L1133 (98.973, 52.509) -> (97.974, 52.509)
  line L1134 (183.673, -18.7426) -> (183.673, -15.9426)
  line L1135 (90.031, 80.0836) -> (90.031, 76.9844)
  line L1136 (76.256, 96.6592) -> (77.055, 96.6592)
  line L1137 (98.204, 55.7585) -> (97.224, 55.7585)
  line L1138 (98.973, 53.3084) -> (102.073, 53.3084)
  line L1139 (104.474, 60.7841) -> (104.474, 61.6082)
  line L1140 (90.031, 80.0836) -> (90.83, 80.0836)
  line L1141 (138.167, 99.7592) -> (138.167, 105.5592)
  line L1142 (62.255, 105.5592) -> (62.255, 99.7592)
  line L1143 (98.973, 53.3084) -> (98.973, 52.509)
  line L1144 (138.167, 96.6592) -> (138.167, 95.6582)
  line L1145 (143.217, 95.6582) -> (143.217, 96.6592)
  line L1146 (77.055, 105.5592) -> (76.256, 105.5592)
  line L1147 (222.567, -13.9426) -> (185.673, -13.9426)
  line L1148 (76.256, 109.6602) -> (62.255, 109.6602)
  line L1149 (89.306, 79.6137) -> (89.306, 76.3836)
  line L1150 (-86.2521, 4.3343) -> (-89.551, 4.3343)
  line L1151 (87.581, 79.6137) -> (87.581, 80.5344)
  line L1152 (76.256, 95.6582) -> (62.255, 95.6582)
  line L1153 (142.417, 99.7592) -> (142.417, 96.6592)
  line L1154 (77.055, 108.6602) -> (77.055, 105.5592)
  line L1155 (62.255, 95.6582) -> (76.256, 95.6582)
  line L1156 (97.224, 59.0591) -> (97.224, 55.7585)
  line L1157 (138.968, 96.6592) -> (138.167, 96.6592)
  line L1158 (84.28, 80.5344) -> (87.581, 80.5344)
  line L1159 (138.968, 99.7592) -> (138.167, 99.7592)
  line L1160 (171.573, -20.7426) -> (172.373, -20.7426)
  line L1161 (86.58, 57.9344) -> (86.58, 61.0336)
  line L1162 (138.968, 52.1344) -> (138.968, 49.0338)
  line L1163 (85.781, 52.1344) -> (85.781, 57.9344)
  line L1164 (124.167, 105.5592) -> (124.167, 99.7592)
  line L1165 (99.556, 96.6592) -> (99.556, 99.7592)
  line L1166 (143.217, 49.0338) -> (142.417, 49.0338)
  line L1167 (114.356, 95.6582) -> (100.355, 95.6582)
  line L1168 (110.503, 60.7841) -> (110.503, 59.0591)
  line L1169 (37.642, 38.8844) -> (38.442, 38.8844)
  line L1170 (86.58, 52.1344) -> (86.58, 49.0338)
  line L1171 (138.968, 57.9344) -> (138.968, 61.0336)
  line L1172 (100.355, 99.7592) -> (99.556, 99.7592)
  line L1173 (124.167, 96.6592) -> (123.367, 96.6592)
  line L1174 (138.968, 57.9344) -> (138.167, 57.9344)
  line L1175 (85.781, 48.0333) -> (85.781, 49.0338)
  line L1176 (111.423, 55.7585) -> (110.503, 55.7585)
  line L1177 (85.781, 57.9344) -> (85.781, 52.1344)
  line L1178 (115.155, 99.7592) -> (114.356, 99.7592)
  line L1179 (100.355, 105.5592) -> (100.355, 99.7592)
  line L1180 (38.442, 33.0844) -> (38.442, 38.8844)
  line L1181 (33.392, 38.8844) -> (33.392, 33.0844)
  line L1182 (33.392, 41.9836) -> (33.392, 42.984)
  line L1183 (138.167, 61.0336) -> (138.167, 62.034)
  line L1184 (37.642, 29.9838) -> (37.642, 33.0844)
  line L1185 (85.781, 57.9344) -> (86.58, 57.9344)
  line L1186 (85.781, 61.0336) -> (85.781, 62.034)
  line L1187 (111.973, 52.509) -> (110.974, 52.509)
  line L1188 (143.217, 48.0333) -> (143.217, 49.0338)
  line L1189 (100.355, 96.6592) -> (99.556, 96.6592)
  line L1190 (85.781, 62.034) -> (85.781, 61.0336)
  line L1191 (37.642, 33.0844) -> (38.442, 33.0844)
  line L1192 (114.356, 99.7592) -> (115.155, 99.7592)
  line L1193 (110.974, 52.509) -> (110.974, 53.3084)
  line L1194 (85.781, 61.0336) -> (86.58, 61.0336)
  line L1195 (100.355, 96.6592) -> (100.355, 95.6582)
  line L1196 (110.503, 59.0591) -> (110.503, 60.7841)
  line L1197 (123.367, 99.7592) -> (123.367, 96.6592)
  line L1198 (123.367, 99.7592) -> (124.167, 99.7592)
  line L1199 (138.167, 52.1344) -> (138.968, 52.1344)
  line L1200 (99.556, 99.7592) -> (100.355, 99.7592)
  line L1201 (124.167, 96.6592) -> (124.167, 95.6582)
  line L1202 (123.367, 105.5592) -> (124.167, 105.5592)
  line L1203 (96.105, 99.7592) -> (95.306, 99.7592)
  line L1204 (107.274, 52.509) -> (107.874, 52.509)
  line L1205 (138.167, 62.034) -> (138.167, 61.0336)
  line L1206 (71.78, 62.034) -> (71.78, 61.0336)
  line L1207 (37.642, 33.0844) -> (37.642, 29.9838)
  line L1208 (142.417, 57.9344) -> (143.217, 57.9344)
  line L1209 (114.356, 96.6592) -> (115.155, 96.6592)
  line L1210 (142.417, 52.1344) -> (142.417, 49.0338)
  line L1211 (142.417, 49.0338) -> (142.417, 52.1344)
  line L1212 (114.356, 99.7592) -> (114.356, 105.5592)
  line L1213 (143.217, 52.1344) -> (142.417, 52.1344)
  line L1214 (138.968, 52.1344) -> (138.167, 52.1344)
  line L1215 (38.442, 41.9836) -> (38.442, 42.984)
  line L1216 (100.355, 95.6582) -> (114.356, 95.6582)
  line L1217 (95.306, 96.6592) -> (95.306, 95.6582)
  line L1218 (138.167, 61.0336) -> (138.968, 61.0336)
  line L1219 (143.217, 49.0338) -> (143.217, 48.0333)
  line L1220 (138.167, 57.9344) -> (138.167, 52.1344)
  line L1221 (115.155, 96.6592) -> (115.155, 99.7592)
  line L1222 (96.105, 96.6592) -> (96.105, 99.7592)
  line L1223 (115.155, 96.6592) -> (114.356, 96.6592)
  line L1224 (33.392, 29.9838) -> (34.193, 29.9838)
  line L1225 (33.392, 38.8844) -> (34.193, 38.8844)
  line L1226 (143.217, 57.9344) -> (143.217, 52.1344)
  line L1227 (138.167, 49.0338) -> (138.968, 49.0338)
  line L1228 (71.78, 52.1344) -> (71.78, 57.9344)
  line L1229 (115.155, 99.7592) -> (115.155, 96.6592)
  line L1230 (107.274, 54.0334) -> (110.503, 54.0334)
  line L1231 (114.356, 95.6582) -> (114.356, 96.6592)
  line L1232 (70.981, 61.0336) -> (70.981, 57.9344)
  line L1233 (70.981, 57.9344) -> (71.78, 57.9344)
  line L1234 (33.392, 33.0844) -> (34.193, 33.0844)
  line L1235 (95.306, 105.5592) -> (95.306, 99.7592)
  line L1236 (107.874, 53.3084) -> (110.974, 53.3084)
  line L1237 (38.442, 41.9836) -> (37.642, 41.9836)
  line L1238 (107.274, 61.6082) -> (107.274, 60.7841)
  line L1239 (96.105, 99.7592) -> (96.105, 96.6592)
  line L1240 (71.78, 49.0338) -> (71.78, 48.0333)
  line L1241 (37.642, 29.9838) -> (38.442, 29.9838)
  line L1242 (107.874, 52.509) -> (107.874, 53.3084)
  line L1243 (143.217, 57.9344) -> (142.417, 57.9344)
  line L1244 (143.217, 52.1344) -> (143.217, 57.9344)
  line L1245 (34.193, 33.0844) -> (34.193, 29.9838)
  line L1246 (110.503, 54.0334) -> (110.503, 55.7585)
  line L1247 (70.981, 49.0338) -> (71.78, 49.0338)
  line L1248 (33.392, 41.9836) -> (34.193, 41.9836)
  line L1249 (95.306, 99.7592) -> (96.105, 99.7592)
  line L1250 (70.981, 52.1344) -> (71.78, 52.1344)
  line L1251 (143.217, 61.0336) -> (142.417, 61.0336)
  line L1252 (138.167, 67.0833) -> (124.167, 67.0833)
  line L1253 (95.306, 95.6582) -> (95.306, 96.6592)
  line L1254 (124.167, 67.0833) -> (124.167, 68.0838)
  line L1255 (142.417, 61.0336) -> (143.217, 61.0336)
  line L1256 (124.167, 68.0838) -> (124.167, 67.0833)
  line L1257 (124.167, 109.6602) -> (138.167, 109.6602)
  line L1258 (34.193, 33.0844) -> (33.392, 33.0844)
  line L1259 (71.78, 49.0338) -> (70.981, 49.0338)
  line L1260 (33.392, 28.9833) -> (33.392, 29.9838)
  line L1261 (71.78, 52.1344) -> (70.981, 52.1344)
  line L1262 (38.442, 29.9838) -> (38.442, 28.9833)
  line L1263 (138.167, 95.6582) -> (124.167, 95.6582)
  line L1264 (143.217, 61.0336) -> (143.217, 62.034)
  line L1265 (37.642, 41.9836) -> (38.442, 41.9836)
  line L1266 (107.274, 61.6082) -> (104.474, 61.6082)
  line L1267 (124.167, 81.084) -> (138.167, 81.084)
  line L1268 (71.78, 61.0336) -> (71.78, 62.034)
  line L1269 (124.167, 68.0838) -> (123.367, 68.0838)
  line L1270 (70.981, 49.0338) -> (70.981, 52.1344)
  line L1271 (-90.1451, 95.6582) -> (-76.144, 95.6582)
  line L1272 (142.417, 49.0338) -> (143.217, 49.0338)
  line L1273 (138.968, 61.0336) -> (138.968, 57.9344)
  line L1274 (34.193, 38.8844) -> (34.193, 41.9836)
  line L1275 (124.167, 48.0333) -> (138.167, 48.0333)
  line L1276 (71.78, 57.9344) -> (70.981, 57.9344)
  line L1277 (110.503, 54.0334) -> (107.274, 54.0334)
  line L1278 (34.193, 41.9836) -> (33.392, 41.9836)
  line L1279 (104.474, 61.6082) -> (107.274, 61.6082)
  line L1280 (71.78, 61.0336) -> (70.981, 61.0336)
  line L1281 (70.981, 52.1344) -> (70.981, 49.0338)
  line L1282 (70.981, 61.0336) -> (71.78, 61.0336)
  line L1283 (85.781, 48.0333) -> (71.78, 48.0333)
  line L1284 (124.167, 81.084) -> (124.167, 80.0836)
  line L1285 (38.442, 28.9833) -> (38.442, 29.9838)
  line L1286 (123.367, 76.9844) -> (124.167, 76.9844)
  line L1287 (123.367, 71.1844) -> (124.167, 71.1844)
  line L1288 (124.167, 71.1844) -> (124.167, 76.9844)
  line L1289 (138.167, 48.0333) -> (124.167, 48.0333)
  line L1290 (110.503, 59.0591) -> (111.423, 59.0591)
  line L1291 (70.981, 57.9344) -> (70.981, 61.0336)
  line L1292 (123.367, 71.1844) -> (123.367, 68.0838)
  line L1293 (123.367, 80.0836) -> (123.367, 76.9844)
  line L1294 (33.392, 29.9838) -> (33.392, 28.9833)
  line L1295 (33.392, 42.984) -> (33.392, 41.9836)
  line L1296 (85.781, 62.034) -> (71.78, 62.034)
  line L1297 (261.656, 114.1832) -> (261.656, -13.9426)
  line L1298 (107.874, 53.3084) -> (107.874, 52.509)
  line L1299 (110.503, 60.7841) -> (107.274, 60.7841)
  line L1300 (111.423, 59.0591) -> (110.503, 59.0591)
  line L1301 (138.167, 62.034) -> (124.167, 62.034)
  line L1302 (124.167, 62.034) -> (138.167, 62.034)
  line L1303 (124.167, 67.0833) -> (138.167, 67.0833)
  line L1304 (111.423, 55.7585) -> (111.423, 59.0591)
  line L1305 (34.193, 41.9836) -> (34.193, 38.8844)
  line L1306 (34.193, 29.9838) -> (33.392, 29.9838)
  line L1307 (110.503, 55.7585) -> (110.503, 54.0334)
  line L1308 (107.274, 54.0334) -> (107.274, 52.509)
  line L1309 (107.274, 60.7841) -> (110.503, 60.7841)
  line L1310 (76.256, 81.084) -> (62.255, 81.084)
  line L1311 (33.392, 33.0844) -> (33.392, 38.8844)
  line L1312 (71.78, 48.0333) -> (85.781, 48.0333)
  line L1313 (38.442, 42.984) -> (38.442, 41.9836)
  line L1314 (34.193, 29.9838) -> (34.193, 33.0844)
  line L1315 (71.78, 62.034) -> (85.781, 62.034)
  line L1316 (124.167, 71.1844) -> (123.367, 71.1844)
  line L1317 (138.167, 67.0833) -> (138.167, 68.0838)
  line L1318 (123.367, 68.0838) -> (124.167, 68.0838)
  line L1319 (110.503, 55.7585) -> (111.423, 55.7585)
  line L1320 (99.556, 108.6602) -> (100.355, 108.6602)
  line L1321 (81.305, 105.5592) -> (81.305, 99.7592)
  line L1322 (138.167, 109.6602) -> (124.167, 109.6602)
  line L1323 (34.193, 38.8844) -> (33.392, 38.8844)
  line L1324 (123.367, 76.9844) -> (123.367, 80.0836)
  line L1325 (124.167, 95.6582) -> (138.167, 95.6582)
  line L1326 (114.356, 108.6602) -> (115.155, 108.6602)
  line L1327 (107.274, 60.7841) -> (107.274, 61.6082)
  line L1328 (90.83, 67.0833) -> (104.831, 67.0833)
  line L1329 (38.442, 33.0844) -> (37.642, 33.0844)
  line L1330 (124.167, 80.0836) -> (123.367, 80.0836)
  line L1331 (100.355, 105.5592) -> (99.556, 105.5592)
  line L1332 (80.506, 108.6602) -> (81.305, 108.6602)
  line L1333 (138.167, 81.084) -> (124.167, 81.084)
  line L1334 (124.167, 76.9844) -> (123.367, 76.9844)